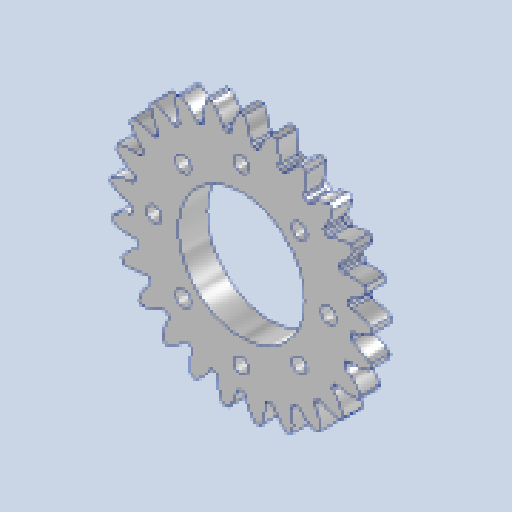
# Autodesk Inventor part: 기어1
Saved by Autodesk Inventor 2023.1 (Build 271208000, 208)
## iProperties
Created: 2022-10-17
Part Number: 기어1
Material: 알루미늄 6061
Document SubType Name: Modeling
Designer: BAEK
Density: 2.7 g/cm^3
Appearance: 알루미늄 - 평지
Mass: 32.3459 g
Surface Area: 83.0255 cm^2
Volume: 11.98 cm^3
Author: BAEK
Autodesk Inventor part; units mm, degrees
ref_plane "YZ Plane" through (0, 0, 0) normal (1, 0, 0) x (0, 1, 0)
ref_plane "XZ Plane" through (0, 0, 0) normal (0, 1, 0) x (-1, 0, 0)
ref_plane "XY Plane" through (0, 0, 0) normal (0, 0, 1) x (1, 0, 0)
sketch "스케치1" plane through (0, 0, 0) normal (0, 0, 1) x (1, 0, 0)
  circle A0 centre (0, 0) radius 25 construction
  circle A1 centre (0, 0) radius 27 construction
  arc A2 (-2.4811, 22.3628) -> (2.4811, 22.3628) centre (0, 0) ccw
  line L0 (0, 0) -> (0, 27) construction
  line L1 (-0.57, 0) -> (-0.57, 26.994) construction
  line L2 (-1.57, 0) -> (-1.57, 26.9543) construction
  line L3 (-2.07, 0) -> (-2.07, 26.9205) construction
  arc A3 (-0.57, 26.994) -> (-2.0388, 22.8087) centre (7.4248, 21.8379) ccw
  arc A4 (2.0388, 22.8087) -> (0.57, 26.994) centre (-7.4248, 21.8379) ccw
  line L4 (-0.57, 26.994) -> (0.57, 26.994)
  arc A5 (-2.4811, 22.3628) -> (-2.0388, 22.8087) centre (-2.5362, 22.8597) ccw
  arc A6 (2.0388, 22.8087) -> (2.4811, 22.3628) centre (2.5362, 22.8597) ccw
  dimension "d0" = 50
  dimension "d1" = 2
  dimension "d2" = 4.5
  dimension "d3" = 0.5
  dimension "d4" = 1
  dimension "d6" = 1.57
  dimension "d7" = 0.5
  constraints: 14 point on circle, 10 end point, 7 centre point, 4 tangent, 4 vertical, 3 coincident, 2 symmetric about line, 1 equal radius, 1 horizontal, 1 other
  measures "d0" diameter of A0
  measures "d1" radial gap between concentric circles of A1 A0
  measures "d2" radial gap between concentric circles of A1 A2
  measures "d3" distance between parallel lines of L2 L3
  measures "d4" distance between parallel lines of L1 L2
  measures "d6" distance between parallel lines of L2 L0
  measures "d7" radius of A5
extrude "돌출1" add sketch "스케치1" along normal blind 4
pattern_circular "원형 패턴1" count 25 over 360 about axis through (0, 0, 0) along (0, 0, 1) of "돌출1"
sketch "스케치2" plane through (0, 0, 4) normal (0, 0, 1) x (1, 0, 0)
  line L0 (-9, 43) -> (9, 43)
  arc A0 (12, 40) -> (9, 43) centre (9, 40) ccw
  line L1 (12, 40) -> (12, 32)
  arc A1 (9, 29) -> (12, 32) centre (9, 32) ccw
  line L2 (9, 29) -> (-9, 29)
  arc A2 (-12, 32) -> (-9, 29) centre (-9, 32) ccw
  line L3 (-12, 32) -> (-12, 40)
  arc A3 (-9, 43) -> (-12, 40) centre (-9, 40) ccw
  arc A4 (27, 57) -> (22, 62) centre (22, 57) ccw
  line L4 (22, 62) -> (-22, 62)
  arc A5 (-22, 62) -> (-27, 57) centre (-22, 57) ccw
  line L5 (-27, 57) -> (-27, 55)
  line L6 (-27, 55) -> (-23, 0)
  arc A6 (-23, 0) -> (23, 0) centre (0, 0) ccw
  line L7 (23, 0) -> (27, 55)
  line L8 (27, 55) -> (27, 57)
  circle A7 centre (9, 57.5) radius 1.6
  circle A8 centre (18, 57.5) radius 1.6
  circle A9 centre (0, 57.5) radius 1.6
  circle A10 centre (-18, 57.5) radius 1.6
  circle A11 centre (-9, 57.5) radius 1.6
  circle A12 centre (0, 18) radius 1.6
  circle A13 centre (12, 12) radius 1.6
  circle A14 centre (-12, 12) radius 1.6
  circle A15 centre (-18, 0) radius 1.6
  circle A16 centre (12, -12) radius 1.6
  circle A17 centre (0, -18) radius 1.6
  circle A18 centre (-12, -12) radius 1.6
  circle A19 centre (18, 0) radius 1.6
  circle A20 centre (0, 0) radius 13
  circle A21 centre (0, 0) radius 23
  constraints: 22 centre point, 18 end point, 14 point on circle, 1 coincident, 1 concentric
extrude "돌출2" cut sketch "스케치2" against normal blind 10 contours A12 | A13 | A14 | A15 | A16 | A17 | A18 | A19 | A20
sketch "스케치3" plane through (0, 0, 0) normal (0, 0, -1) x (-1, 0, 0)
  circle A0 centre (0, 0) radius 21
  circle A1 centre (12, 12) radius 1.6 projected
  circle A2 centre (0, -18) radius 1.6 projected
  circle A3 centre (-18, 0) radius 1.6 projected
  circle A4 centre (18, 0) radius 1.6 projected
  circle A5 centre (0, 18) radius 1.6 projected
  circle A6 centre (-12, -12) radius 1.6 projected
  circle A7 centre (-12, 12) radius 1.6 projected
  circle A8 centre (12, -12) radius 1.6 projected
  circle A9 centre (0, 0) radius 13 projected
  arc A10 (2.0388, 22.8087) -> (2.4811, 22.3628) centre (2.5362, 22.8597) ccw projected
  arc A11 (2.0388, 22.8087) -> (0.57, 26.994) centre (-7.4248, 21.8379) ccw projected
  line L0 (-0.57, 26.994) -> (0.57, 26.994) projected
  arc A12 (-0.57, 26.994) -> (-2.0388, 22.8087) centre (7.4248, 21.8379) ccw projected
  arc A13 (-2.4811, 22.3628) -> (-2.0388, 22.8087) centre (-2.5362, 22.8597) ccw projected
  arc A14 (-2.4811, 22.3628) -> (-3.1583, 22.2772) centre (0, 0) ccw projected
  arc A15 (-3.6975, 22.5992) -> (-3.1583, 22.2772) centre (-3.2285, 22.7723) ccw projected
  arc A16 (-3.6975, 22.5992) -> (-6.161, 26.2877) centre (-12.6224, 19.3053) ccw projected
  line L1 (-7.2652, 26.0042) -> (-6.161, 26.2877) projected
  arc A17 (-7.2652, 26.0042) -> (-7.647, 21.5851) centre (1.7607, 22.9983) ccw projected
  arc A18 (-7.9645, 21.0432) -> (-7.647, 21.5851) centre (-8.1415, 21.5108) ccw projected
  arc A19 (-7.9645, 21.0432) -> (-8.5992, 20.7919) centre (0, 0) ccw projected
  arc A20 (-9.2016, 20.9696) -> (-8.5992, 20.7919) centre (-8.7903, 21.254) ccw projected
  arc A21 (-9.2016, 20.9696) -> (-12.505, 23.9296) centre (-17.0269, 15.5597) ccw projected
  line L2 (-13.5039, 23.3804) -> (-12.505, 23.9296) projected
  arc A22 (-13.5039, 23.3804) -> (-12.7748, 19.0052) centre (-4.014, 22.7136) ccw projected
  arc A23 (-12.9475, 18.4014) -> (-12.7748, 19.0052) centre (-13.2352, 18.8103) ccw projected
  arc A24 (-12.9475, 18.4014) -> (-13.4998, 18.0002) centre (0, 0) ccw projected
  arc A25 (-14.1274, 18.0225) -> (-13.4998, 18.0002) centre (-13.7998, 18.4002) ccw projected
  arc A26 (-14.1274, 18.0225) -> (-18.0631, 20.068) centre (-20.3615, 10.8365) ccw projected
  line L3 (-18.8942, 19.2876) -> (-18.0631, 20.068) projected
  arc A27 (-18.8942, 19.2876) -> (-17.0999, 15.2312) centre (-9.5366, 21.0018) ccw projected
  arc A28 (-17.117, 14.6034) -> (-17.0999, 15.2312) centre (-17.4974, 14.9279) ccw projected
  arc A29 (-17.117, 14.6034) -> (-17.5521, 14.0774) centre (0, 0) ccw projected
  arc A30 (-18.1656, 13.9429) -> (-17.5521, 14.0774) centre (-17.9422, 14.3902) ccw projected
  arc A31 (-18.1656, 13.9429) -> (-22.4864, 14.9454) centre (-22.4167, 5.4323) ccw projected
  line L4 (-23.0972, 13.9828) -> (-22.4864, 14.9454) projected
  arc A32 (-23.0972, 13.9828) -> (-20.3505, 10.5001) centre (-14.4599, 17.9703) ccw projected
  arc A33 (-20.2109, 9.8878) -> (-20.3505, 10.5001) centre (-20.6601, 10.1075) ccw projected
  arc A34 (-20.2109, 9.8878) -> (-20.5016, 9.2701) centre (0, 0) ccw projected
  arc A35 (-21.0624, 8.9873) -> (-20.5016, 9.2701) centre (-20.9572, 9.4761) ccw projected
  arc A36 (-21.0624, 8.9873) -> (-25.4967, 8.8837) centre (-23.0634, -0.3132) ccw projected
  line L5 (-25.8489, 7.7995) -> (-25.4967, 8.8837) projected
  arc A37 (-25.8489, 7.7995) -> (-22.3224, 5.1093) centre (-18.4746, 13.8097) ccw projected
  arc A38 (-22.035, 4.5509) -> (-22.3224, 5.1093) centre (-22.5246, 4.652) ccw projected
  arc A39 (-22.035, 4.5509) -> (-22.1629, 3.8803) centre (0, 0) ccw projected
  arc A40 (-22.6357, 3.467) -> (-22.1629, 3.8803) centre (-22.6554, 3.9666) ccw projected
  arc A41 (-22.6357, 3.467) -> (-26.9049, 2.2638) centre (-22.261, -6.039) ccw projected
  line L6 (-26.9765, 1.1261) -> (-26.9049, 2.2638) projected
  arc A42 (-26.9765, 1.1261) -> (-22.8917, -0.6026) centre (-21.3286, 8.7814) ccw projected
  arc A43 (-22.4744, -1.072) -> (-22.8917, -0.6026) centre (-22.9739, -1.0958) ccw projected
  arc A44 (-22.4744, -1.072) -> (-22.4316, -1.7533) centre (0, 0) ccw projected
  arc A45 (-22.7867, -2.2712) -> (-22.4316, -1.7533) centre (-22.9301, -1.7922) ccw projected
  arc A46 (-22.7867, -2.2712) -> (-26.6227, -4.4983) centre (-20.0598, -11.3853) ccw projected
  line L7 (-26.409, -5.6181) -> (-26.6227, -4.4983) projected
  arc A47 (-26.409, -5.6181) -> (-22.0227, -6.2766) centre (-22.8423, 3.2013) ccw projected
  arc A48 (-21.5018, -6.6275) -> (-22.0227, -6.2766) centre (-21.9796, -6.7748) ccw projected
  arc A49 (-21.5018, -6.6275) -> (-21.2908, -7.2767) centre (0, 0) ccw projected
  arc A50 (-21.506, -7.8667) -> (-21.2908, -7.2767) centre (-21.764, -7.4384) ccw projected
  arc A51 (-21.506, -7.8667) -> (-24.6676, -10.9777) centre (-16.5981, -16.0163) ccw projected
  line L8 (-24.1822, -12.0092) -> (-24.6676, -10.9777) projected
  arc A52 (-24.1822, -12.0092) -> (-19.7699, -11.5562) centre (-22.9208, -2.5799) ccw projected
  arc A53 (-19.1781, -11.7665) -> (-19.7699, -11.5562) centre (-19.6043, -12.028) ccw projected
  arc A54 (-19.1781, -11.7665) -> (-18.8123, -12.3429) centre (0, 0) ccw projected
  arc A55 (-18.874, -12.9679) -> (-18.8123, -12.3429) centre (-19.2304, -12.6172) ccw projected
  arc A56 (-18.874, -12.9679) -> (-21.1626, -16.7674) centre (-12.0936, -19.6409) ccw projected
  line L9 (-20.4359, -17.6458) -> (-21.1626, -16.7674) projected
  arc A57 (-20.4359, -17.6458) -> (-16.2748, -16.1097) centre (-21.5591, -8.199) ccw projected
  arc A58 (-15.6493, -16.1663) -> (-16.2748, -16.1097) centre (-15.9971, -16.5255) ccw projected
  arc A59 (-15.6493, -16.1663) -> (-15.1517, -16.6335) centre (0, 0) ccw projected
  arc A60 (-15.0561, -17.2543) -> (-15.1517, -16.6335) centre (-15.4884, -17.0032) ccw projected
  arc A61 (-15.0561, -17.2543) -> (-16.3278, -21.5036) centre (-6.8292, -22.0314) ccw projected
  line L10 (-15.4055, -22.1736) -> (-16.3278, -21.5036) projected
  arc A62 (-15.4055, -22.1736) -> (-11.7572, -19.651) centre (-18.8428, -13.303) ccw projected
  arc A63 (-11.1373, -19.5502) -> (-11.7572, -19.651) centre (-11.3848, -19.9847) ccw projected
  arc A64 (-11.1373, -19.5502) -> (-10.5391, -19.8791) centre (0, 0) ccw projected
  arc A65 (-10.2921, -20.4565) -> (-10.5391, -19.8791) centre (-10.7733, -20.3208) ccw projected
  arc A66 (-10.2921, -20.4565) -> (-10.4671, -24.8885) centre (-1.1356, -23.0376) ccw projected
  line L11 (-9.4072, -25.3082) -> (-10.4671, -24.8885) projected
  arc A67 (-9.4072, -25.3082) -> (-6.5008, -21.9575) centre (-14.9425, -17.5711) ccw projected
  arc A68 (-5.9255, -21.7057) -> (-6.5008, -21.9575) centre (-6.0571, -22.1881) ccw projected
  arc A69 (-5.9255, -21.7057) -> (-5.2643, -21.8755) centre (0, 0) ccw projected
  arc A70 (-4.8814, -22.3733) -> (-5.2643, -21.8755) centre (-5.3813, -22.3616) ccw projected
  arc A71 (-4.8814, -22.3733) -> (-3.9487, -26.7097) centre (4.6293, -22.5962) ccw projected
  line L12 (-2.8177, -26.8526) -> (-3.9487, -26.7097) projected
  arc A72 (-2.8177, -26.8526) -> (-0.836, -22.8844) centre (-10.1033, -20.7351) ccw projected
  arc A73 (-0.3413, -22.4974) -> (-0.836, -22.8844) centre (-0.3489, -22.9974) ccw projected
  arc A74 (-0.3413, -22.4974) -> (0.3413, -22.4974) centre (0, 0) ccw projected
  arc A75 (0.836, -22.8844) -> (0.3413, -22.4974) centre (0.3489, -22.9974) ccw projected
  arc A76 (0.836, -22.8844) -> (2.8177, -26.8526) centre (10.1033, -20.7351) ccw projected
  line L13 (3.9487, -26.7097) -> (2.8177, -26.8526) projected
  arc A77 (3.9487, -26.7097) -> (4.8814, -22.3733) centre (-4.6293, -22.5962) ccw projected
  arc A78 (5.2643, -21.8755) -> (4.8814, -22.3733) centre (5.3813, -22.3616) ccw projected
  arc A79 (5.2643, -21.8755) -> (5.9255, -21.7057) centre (0, 0) ccw projected
  arc A80 (6.5008, -21.9575) -> (5.9255, -21.7057) centre (6.0571, -22.1881) ccw projected
  arc A81 (6.5008, -21.9575) -> (9.4072, -25.3082) centre (14.9425, -17.5711) ccw projected
  line L14 (10.4671, -24.8885) -> (9.4072, -25.3082) projected
  arc A82 (10.4671, -24.8885) -> (10.2921, -20.4565) centre (1.1356, -23.0376) ccw projected
  arc A83 (10.5391, -19.8791) -> (10.2921, -20.4565) centre (10.7733, -20.3208) ccw projected
  arc A84 (10.5391, -19.8791) -> (11.1373, -19.5502) centre (0, 0) ccw projected
  arc A85 (11.7572, -19.651) -> (11.1373, -19.5502) centre (11.3848, -19.9847) ccw projected
  arc A86 (11.7572, -19.651) -> (15.4055, -22.1736) centre (18.8428, -13.303) ccw projected
  line L15 (16.3278, -21.5036) -> (15.4055, -22.1736) projected
  arc A87 (16.3278, -21.5036) -> (15.0561, -17.2543) centre (6.8292, -22.0314) ccw projected
  arc A88 (15.1517, -16.6335) -> (15.0561, -17.2543) centre (15.4884, -17.0032) ccw projected
  arc A89 (15.1517, -16.6335) -> (15.6493, -16.1663) centre (0, 0) ccw projected
  arc A90 (16.2748, -16.1097) -> (15.6493, -16.1663) centre (15.9971, -16.5255) ccw projected
  arc A91 (16.2748, -16.1097) -> (20.4359, -17.6458) centre (21.5591, -8.199) ccw projected
  line L16 (21.1626, -16.7674) -> (20.4359, -17.6458) projected
  arc A92 (21.1626, -16.7674) -> (18.874, -12.9679) centre (12.0936, -19.6409) ccw projected
  arc A93 (18.8123, -12.3429) -> (18.874, -12.9679) centre (19.2304, -12.6172) ccw projected
  arc A94 (18.8123, -12.3429) -> (19.1781, -11.7665) centre (0, 0) ccw projected
  arc A95 (19.7699, -11.5562) -> (19.1781, -11.7665) centre (19.6043, -12.028) ccw projected
  arc A96 (19.7699, -11.5562) -> (24.1822, -12.0092) centre (22.9208, -2.5799) ccw projected
  line L17 (24.6676, -10.9777) -> (24.1822, -12.0092) projected
  arc A97 (24.6676, -10.9777) -> (21.506, -7.8667) centre (16.5981, -16.0163) ccw projected
  arc A98 (21.2908, -7.2767) -> (21.506, -7.8667) centre (21.764, -7.4384) ccw projected
  arc A99 (21.2908, -7.2767) -> (21.5018, -6.6275) centre (0, 0) ccw projected
  arc A100 (22.0227, -6.2766) -> (21.5018, -6.6275) centre (21.9796, -6.7748) ccw projected
  arc A101 (22.0227, -6.2766) -> (26.409, -5.6181) centre (22.8423, 3.2013) ccw projected
  line L18 (26.6227, -4.4983) -> (26.409, -5.6181) projected
  arc A102 (26.6227, -4.4983) -> (22.7867, -2.2712) centre (20.0598, -11.3853) ccw projected
  arc A103 (22.4316, -1.7533) -> (22.7867, -2.2712) centre (22.9301, -1.7922) ccw projected
  arc A104 (22.4316, -1.7533) -> (22.4744, -1.072) centre (0, 0) ccw projected
  arc A105 (22.8917, -0.6026) -> (22.4744, -1.072) centre (22.9739, -1.0958) ccw projected
  arc A106 (22.8917, -0.6026) -> (26.9765, 1.1261) centre (21.3286, 8.7814) ccw projected
  line L19 (26.9049, 2.2638) -> (26.9765, 1.1261) projected
  arc A107 (26.9049, 2.2638) -> (22.6357, 3.467) centre (22.261, -6.039) ccw projected
  arc A108 (22.1629, 3.8803) -> (22.6357, 3.467) centre (22.6554, 3.9666) ccw projected
  arc A109 (22.1629, 3.8803) -> (22.035, 4.5509) centre (0, 0) ccw projected
  arc A110 (22.3224, 5.1093) -> (22.035, 4.5509) centre (22.5246, 4.652) ccw projected
  arc A111 (22.3224, 5.1093) -> (25.8489, 7.7995) centre (18.4746, 13.8097) ccw projected
  line L20 (25.4967, 8.8837) -> (25.8489, 7.7995) projected
  arc A112 (25.4967, 8.8837) -> (21.0624, 8.9873) centre (23.0634, -0.3132) ccw projected
  arc A113 (20.5016, 9.2701) -> (21.0624, 8.9873) centre (20.9572, 9.4761) ccw projected
  arc A114 (20.5016, 9.2701) -> (20.2109, 9.8878) centre (0, 0) ccw projected
  arc A115 (20.3505, 10.5001) -> (20.2109, 9.8878) centre (20.6601, 10.1075) ccw projected
  arc A116 (20.3505, 10.5001) -> (23.0972, 13.9828) centre (14.4599, 17.9703) ccw projected
  line L21 (22.4864, 14.9454) -> (23.0972, 13.9828) projected
  arc A117 (22.4864, 14.9454) -> (18.1656, 13.9429) centre (22.4167, 5.4323) ccw projected
  arc A118 (17.5521, 14.0774) -> (18.1656, 13.9429) centre (17.9422, 14.3902) ccw projected
  arc A119 (17.5521, 14.0774) -> (17.117, 14.6034) centre (0, 0) ccw projected
  arc A120 (17.0999, 15.2312) -> (17.117, 14.6034) centre (17.4974, 14.9279) ccw projected
  arc A121 (17.0999, 15.2312) -> (18.8942, 19.2876) centre (9.5366, 21.0018) ccw projected
  line L22 (18.0631, 20.068) -> (18.8942, 19.2876) projected
  arc A122 (18.0631, 20.068) -> (14.1274, 18.0225) centre (20.3615, 10.8365) ccw projected
  arc A123 (13.4998, 18.0002) -> (14.1274, 18.0225) centre (13.7998, 18.4002) ccw projected
  arc A124 (13.4998, 18.0002) -> (12.9475, 18.4014) centre (0, 0) ccw projected
  arc A125 (12.7748, 19.0052) -> (12.9475, 18.4014) centre (13.2352, 18.8103) ccw projected
  arc A126 (12.7748, 19.0052) -> (13.5039, 23.3804) centre (4.014, 22.7136) ccw projected
  line L23 (12.505, 23.9296) -> (13.5039, 23.3804) projected
  arc A127 (12.505, 23.9296) -> (9.2016, 20.9696) centre (17.0269, 15.5597) ccw projected
  arc A128 (8.5992, 20.7919) -> (9.2016, 20.9696) centre (8.7903, 21.254) ccw projected
  arc A129 (8.5992, 20.7919) -> (7.9645, 21.0432) centre (0, 0) ccw projected
  arc A130 (7.647, 21.5851) -> (7.9645, 21.0432) centre (8.1415, 21.5108) ccw projected
  arc A131 (7.647, 21.5851) -> (7.2652, 26.0042) centre (-1.7607, 22.9983) ccw projected
  line L24 (6.161, 26.2877) -> (7.2652, 26.0042) projected
  arc A132 (6.161, 26.2877) -> (3.6975, 22.5992) centre (12.6224, 19.3053) ccw projected
  arc A133 (3.1583, 22.2772) -> (3.6975, 22.5992) centre (3.2285, 22.7723) ccw projected
  arc A134 (3.1583, 22.2772) -> (2.4811, 22.3628) centre (0, 0) ccw projected
  dimension "d15" = 42
  constraints: 1 centre point, 1 coincident
  measures "d15" diameter of A0
extrude "돌출3" add sketch "스케치3" along normal blind 2 contours A0
